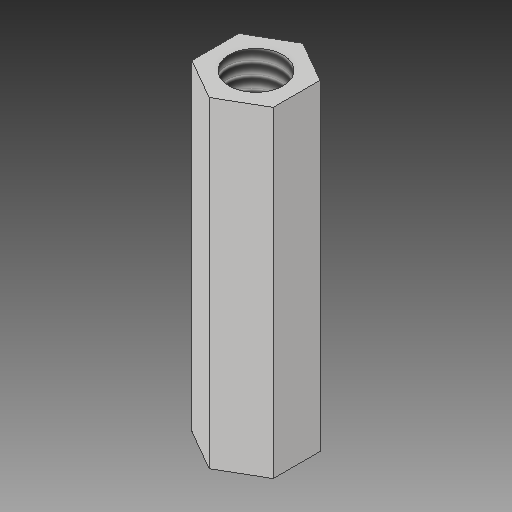
# Autodesk Inventor part: 12mm_M2.5_standoff
Saved by Autodesk Inventor 2018 (Build 220112000, 112)
## iProperties
Created: 2018-05-08
Part Number: 12mm_M2.5_standoff
Material: Generic
Document SubType Name: Modeling
Designer: mmarkle
Density: 1 g/cm^3
Appearance: Default
Author: mmarkle
Autodesk Inventor part; units mm, degrees
ref_plane "YZ Plane" through (0, 0, 0) normal (1, 0, 0) x (0, 1, 0)
ref_plane "XZ Plane" through (0, 0, 0) normal (0, 1, 0) x (-1, 0, 0)
ref_plane "XY Plane" through (0, 0, 0) normal (0, 0, 1) x (1, 0, 0)
sketch "Sketch1" plane through (0, 0, 0) normal (0, 1, 0) x (-1, 0, 0)
  line L0 (1.5155, -0.875) -> (0, -1.75)
  line L1 (0, -1.75) -> (-1.5155, -0.875)
  line L2 (-1.5155, -0.875) -> (-1.5155, 0.875)
  line L3 (-1.5155, 0.875) -> (0, 1.75)
  line L4 (0, 1.75) -> (1.5155, 0.875)
  line L5 (1.5155, 0.875) -> (1.5155, -0.875)
  point P0 (0, 0)
  point P1 (0, 0)
  dimension "d0" = 1.75
  constraints: 12 end point, 1 coincident, 1 vertical alignment, 13 other
  measures "d0" distance of L0.end point (0, 0)
extrude "Extrusion1" add sketch "Sketch1" along normal blind 12
sketch "Sketch2" plane through (0, 12, 0) normal (0, 1, 0) x (1, 0, 0)
  point P0 (0, 0)
  point P1 (0, 0)
  constraints: 1 coincident
hole "Hole1" at (0, 12, 0) direction (0, -1, 0) diameter 2.013 end through all thread size "M2.5x0.45" class "6H" standard "ANSI Metric M Profile"
sketch "Sketch3" plane through (0, 0, 0) normal (0, -1, 0) x (1, 0, 0)
  point P0 (-34.949, 34.34)
  point P1 (0, 0)
  point P2 (-40.6419, -41.3626)
  point P3 (-75.5909, -7.0226)
sketch "Sketch4" plane through (0, 12, 0) normal (0, 1, 0) x (1, 0, 0)
  point P0 (0, 0)
  point P1 (-34.949, -34.34)
  point P2 (-40.6419, 41.3626)
  point P3 (-75.5909, 7.0226)
body "Solid1"
